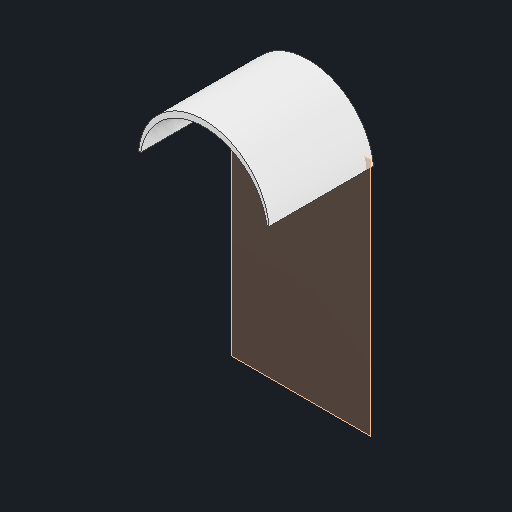
# Autodesk Inventor part: FrontSection2
Saved by Autodesk Inventor 2026.1 (Build 301233000, 233)
## iProperties
Created: 2025-08-01
Part Number: FrontSection2
Material: Plastic, Opaque White
Document SubType Name: Modeling
Designer: Cupri
Density: 0.952 g/cm^3
Appearance: Smooth - White
Author: Cupri
Autodesk Inventor part; units mm, degrees
ref_plane "Work Plane1" through (0, 0, 0) normal (0, 0, 1) x (1, 0, 0)
sketch "Sketch1" plane through (0, 0, 0) normal (0, 0, 1) x (1, 0, 0)
  line L0 (0, 0) -> (145, 0) projected
  line L1 (145, 0) -> (145, 250) projected
  line L2 (0, 250) -> (145, 250) projected
  line L3 (0, 0) -> (0, 250) projected
  line L4 (147.5, 0) -> (-2.5, 0) projected
  line L5 (-2.5, 0) -> (-2.5, 250) projected
  line L6 (147.5, 250) -> (-2.5, 250) projected
  line L7 (147.5, 0) -> (147.5, 250) projected
  arc A0 (145, 250) -> (0, 250) centre (72.5, 238.5041) ccw
  arc A1 (147.5, 250) -> (-2.5, 250) centre (72.5, 243.5041) ccw
  dimension "d0" = 5
  constraints: 4 point on circle, 2 centre point
  measures "d0" distance of A1.centre A0.centre
ref_plane "Work Plane2" through (145, 0, 117.0759) normal (0, 0, 1) x (1, 0, 0)
ref_plane "Work Plane4" through (140, 0, 112.0759) normal (0, 0, 1) x (1, 0, 0)
extrude "Extrusion1" add sketch "Sketch1" along normal up to surface (112.0759 mm away) contours L6 A1 A0
sketch "Sketch2" plane through (0, 0, 0) normal (0, 0, -1) x (-1, 0, 0)
  line L0 (-147.5, 249.9999) -> (2.5, 249.9999) projected
  line L1 (2.5, 250) -> (0, 250) projected
  arc A0 (2.5, 250) -> (-147.5, 250) centre (-72.5, 243.5041) ccw projected
  arc A1 (0, 250) -> (-145, 250) centre (-72.5, 238.5041) ccw projected
  line L2 (-145, 250) -> (-147.5, 250) projected
  point P0 (0, 0)
  point P1 (2.5, 249.9999)
  point P2 (-147.5, 249.9999)
ref_plane "Work Plane3" through (-2.5, 0, -8) normal (0, 0, -1) x (0, 1, 0)
extrude "Extrusion2" add sketch "Sketch2" along normal up to surface (8 mm away) contours A0 L0 A1
body "Solid1"
